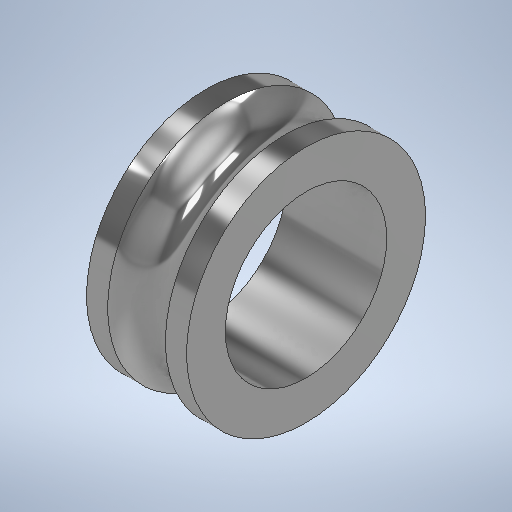
# Autodesk Inventor part: Inner ring
Saved by Autodesk Inventor 2025.1 (Build 291241000, 241)
## iProperties
Created: 2024-08-09
Part Number: Inner ring
Material: Generic
Document SubType Name: Modeling
Designer: vedan
Density: 1 g/cm^3
Appearance: Chrome - Polished Black
Author: vedan
Autodesk Inventor part; units mm, degrees
ref_plane "YZ Plane" through (0, 0, 0) normal (1, 0, 0) x (0, 1, 0)
ref_plane "XY Plane" through (0, 0, 0) normal (0, 0, 1) x (1, 0, 0)
sketch "Sketch2" plane through (0, 0, 0) normal (0, 0, 1) x (1, 0, 0)
  line L0 (-15.5, 25) -> (15.5, 25)
  line L1 (15.5, 25) -> (15.5, 37)
  line L2 (-15.5, 37) -> (-15.5, 25)
  line L3 (-15.5, 25) -> (15.5, 37) construction
  line L4 (15.5, 25) -> (-15.5, 37) construction
  line L5 (0, 0) -> (0, 25) construction
  line L6 (0, 37) -> (0, 45) construction
  arc A0 (-8.9443, 37) -> (8.9443, 37) centre (0, 45) ccw
  line L7 (15.5, 37) -> (8.9443, 37)
  line L8 (-8.9443, 37) -> (-15.5, 37)
  line L9 (-36.1867, 0) -> (33.6957, 0) construction
  point P0 (0, 33)
  dimension "d2" = 12
  dimension "d3" = 25
  dimension "d4" = 8
  dimension "d6" = 12
  dimension "d7" = 31
  constraints: 20 end point, 3 parallel, 3 point on circle, 2 horizontal, 1 centre point, 1 coincident, 1 midpoint, 1 perpendicular, 1 vertical
  measures "d2" distance of L1.end L0.end
  measures "d3" distance of L5.start L5.end
  measures "d4" distance of L6.start L6.end
  measures "d6" distance of point (0, 33) L6.end
  measures "d7" distance of L0.start L0.end
revolve "Revolution1" add sketch "Sketch2" angle 360 about axis through (-36.1867, 0, 0) along (1, 0, 0)
body "Solid1"
